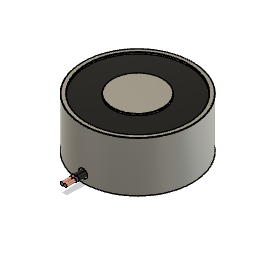
Chess_Board (Autodesk Fusion 360 archive; units mm, degrees)
design "Electromagnet_65x30"
Autodesk Fusion 360 part; units mm, degrees
sketch "Sketch1" plane through (0, 0, 0) normal (0, 1, 0) x (1, 0, 0)
  circle A0 centre (0, 0) radius 32.5
  dimension "d1" = 65
  constraint coincident A0.centre origin
  measures "d1" diameter of A0
extrude "Extrude1" add sketch "Sketch1" along normal blind 30 makes body 1
sketch "Sketch2" plane through (0, 30, 0) normal (0, 1, 0) x (-1, 0, 0)
  circle A0 centre (0, 0) radius 32.5
  circle A1 centre (0, 0) radius 15
  circle A2 centre (0, 0) radius 30
  dimension "d4" = 30
  dimension "d5" = 60
  constraint coincident A0.centre A1.centre
  measures "d4" diameter of A1
  measures "d5" diameter of A2
extrude "Extrude2" cut sketch "Sketch2" against normal blind 1 contours A2 bodies 1
fillet "Fillet1" radius 0.2 4 edges at (13.9849, 30, -5.4242) (27.9698, 30, 10.8485) (-30.3006, 30, 11.7525) (-30.3006, 0, 11.7525) on bodies 1
sketch "Sketch3" plane through (0, 0, 0) normal (0, 0, 1) x (1, 0, 0)
  circle A0 centre (0, 5) radius 2.5
  dimension "d10" = 5
  dimension "d11" = 5
  constraint vertical origin A0.centre
  measures "d10" diameter of A0
  measures "d11" distance of origin A0.centre
extrude "Extrude3" cut sketch "Sketch3" along normal blind 33 bodies 1
fillet "Fillet2" radius 0.1 1 edges at (-2.5, 5, 32.4037) on bodies 1
sketch "Sketch4" plane through (0, 0, 0) normal (0, 0, 1) x (1, 0, 0)
  circle A0 centre (0, 5) radius 2.5
  line L0 (-0.134, 5.5) -> (0.134, 5.5)
  line L1 (-0.134, 4.5) -> (0.134, 4.5)
  arc A1 (-0.134, 5.5) -> (-0.134, 4.5) centre (-1, 5) ccw
  arc A2 (0.134, 4.5) -> (0.134, 5.5) centre (1, 5) ccw
  arc A3 (0, 4.1693) -> (0, 5.8307) centre (1, 5) ccw
  arc A4 (0, 5.8307) -> (0, 4.1693) centre (-1, 5) ccw
  dimension "d16" = 2
  dimension "d17" = 2
  dimension "d18" = 5
  dimension "d19" = 1
  dimension "d20" = 0.5
  dimension "d21" = 0.5
  dimension "d22" = 0.5
  dimension "d23" = 0.3
  constraint tangent A1 A2
  constraint horizontal L0
  measures "d16" diameter of A1
  measures "d17" diameter of A2
  measures "d18" vertical distance of origin A2.centre
  measures "d19" horizontal distance of origin A1.centre
  measures "d20" distance of A1.centre L0
  measures "d21" distance of A2.centre L1
  measures "d22" distance of A1.centre L1
extrude "Extrude4" add sketch "Sketch4" along normal blind 44 contours L0 L1 A1 A2 bodies 1
extrude "Extrude5" add sketch "Sketch4" along normal blind 37 contours A3 A4 bodies 1
sketch "Sketch5" plane through (0, 0, 44) normal (0, 0, 1) x (1, 0, 0)
  arc A0 (-0.134, 5.5) -> (-0.134, 4.5) centre (-1, 5) ccw
  line L0 (-0.134, 4.5) -> (0.134, 4.5)
  arc A1 (0.134, 4.5) -> (0.134, 5.5) centre (1, 5) ccw
  line L1 (0.134, 5.5) -> (-0.134, 5.5)
  circle A2 centre (1, 5) radius 1
  circle A3 centre (-1, 5) radius 1
  constraint concentric A1 A2
  constraint concentric A0 A3
extrude "Extrude6" cut sketch "Sketch5" against normal blind 5 contours L1 A2 A3 | L0 A2 A3 bodies 1
sketch "Sketch6" plane through (0, 0, 37) normal (0, 0, 1) x (1, 0, 0)
  arc A0 (0, 5.8307) -> (0, 4.1693) centre (-1, 5) ccw
  arc A1 (0, 4.1693) -> (0, 5.8307) centre (1, 5) ccw
  arc A2 (0, 4.4321) -> (0, 5.5679) centre (1, 5) ccw
  arc A3 (0, 5.5679) -> (0, 4.4321) centre (-1, 5) ccw
  circle A4 centre (-1, 5) radius 1
  arc A5 (-0.134, 5.5) -> (-0.134, 4.5) centre (-1, 5) ccw
  line L0 (-0.134, 5.5) -> (0.134, 5.5)
  arc A6 (0.134, 4.5) -> (0.134, 5.5) centre (1, 5) ccw
  line L1 (0.134, 4.5) -> (-0.134, 4.5)
  dimension "d30" = -0.15
extrude "Extrude7" add sketch "Sketch6" along normal blind 1.5 contours A2 A3 | A4 L0 A6 L1 bodies 1
sketch "Sketch7" plane through (0, 0, 0) normal (0, -1, 0) x (1, 0, 0)
  circle A0 centre (0, 0) radius 32.3
  circle A1 centre (0, 0) radius 4
  dimension "d33" = 8
  constraint coincident A0.centre A1.centre
  measures "d33" diameter of A1
extrude "Extrude8" cut sketch "Sketch7" against normal blind 12 contours A1 bodies 1 makes body 2 at (-2.3, 4.9998, 25.7575)

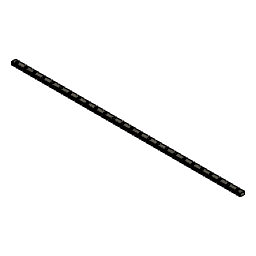
design "MGN12 Rail 650mm"
Autodesk Fusion 360 part; units mm, degrees
sketch "Sketch1" plane through (0, 0, 0) normal (1, 0, 0) x (0, 1, 0)
  line L0 (6, 0) -> (-6, 0)
  line L1 (-6, 8) -> (6, 8)
  line L2 (6, 0) -> (-6, 8) construction
  line L3 (-6, 0) -> (6, 8) construction
  line L4 (5.0369, 5.5) -> (4.7499, 5.5)
  line L5 (4.7499, 5) -> (5.0369, 5)
  line L6 (6, 8) -> (6, 6.245)
  line L7 (6, 4.255) -> (6, 0)
  arc A0 (6, 6.245) -> (5.0369, 5.5) centre (6, 5.25) ccw
  arc A1 (5.0369, 5) -> (6, 4.255) centre (6, 5.25) ccw
  line L8 (0, 8) -> (0, 0) construction
  arc A2 (-5.0369, 5.5) -> (-6, 6.245) centre (-6, 5.25) ccw
  line L9 (-5.0369, 5.5) -> (-4.7499, 5.5)
  line L10 (-4.7499, 5) -> (-5.0369, 5)
  arc A3 (-6, 4.255) -> (-5.0369, 5) centre (-6, 5.25) ccw
  line L11 (-6, 0) -> (-6, 4.255)
  line L12 (-6, 6.245) -> (-6, 8)
  arc A4 (4.7499, 5.5) -> (4.7499, 5) centre (4.7499, 5.25) ccw
  arc A5 (-4.7499, 5) -> (-4.7499, 5.5) centre (-4.7499, 5.25) ccw
  point P0 (0, 4)
  dimension "d1" = 12
  dimension "d2" = 8
  dimension "d6" = 1.99
  dimension "d23" = 1.755
  dimension "d24" = 0.5
  dimension "d25" = 0.287
  constraint perpendicular L0 L11
  constraint parallel L0 L1
  constraint parallel L6 L11
  constraint horizontal L0
  constraint coincident L2 P0
  constraint coincident L3 P0
  constraint midpoint L0 L8.end
  constraint coincident L8.end origin
  constraint perpendicular L4 L6
  constraint perpendicular L5 L6
  constraint coincident A0.centre L6
  constraint coincident L7.start L6
  constraint collinear L6 L7
  constraint coincident L5.end A0
  constraint concentric A0 A1
  constraint midpoint L1 L8.start
  constraint symmetric L7.start L8 A3.start
  constraint symmetric L6.end L8 A2.end
  constraint symmetric L4.start L8 A2.start
  constraint symmetric L5.end L8 L10.end
  constraint symmetric A0 L8 A2
  constraint symmetric A1 L8 A3
  constraint collinear L11 L12
  constraint tangent L4 A4
  constraint tangent L5 A4
  constraint horizontal A0.centre A4.centre
  constraint tangent L10 A5
  constraint tangent L9 A5
  constraint horizontal L9
  constraint horizontal L10
  constraint equal L4 L9
  measures "d1" distance of L0.start L0.end
  measures "d2" distance of L0.start L1.end
  measures "d6" diameter of A0
  measures "d23" distance of L1.end L6.end
  measures "d24" diameter of A4
  measures "d25" distance of L4.start L4.end
extrude "Extrude1" add sketch "Sketch1" along normal blind 650
chamfer "Chamfer1" distance 0.5 angle 45 16 edges at (650, 0, 8) (325, 6, 8) (650, 6, 7.1225) (650, 6, 2.1275) (650, 0, 0) (650, -6, 2.1275) (650, -6, 7.1225) (325, 6, 0) (325, -6, 0) (325, -6, 8) (0, 0, 8) (0, -6, 7.1225) (0, -6, 2.1275) (0, 6, 7.1225) (0, 6, 2.1275) (0, 0, 0)
sketch "Sketch2" plane through (0, 0, 8) normal (0, 0, 1) x (-1, 0, 0)
  line L0 (-0.5, -5.5) -> (-0.5, 5.5)
  line L1 (-0.5, 5.5) -> (-649.5, 5.5)
  line L2 (-649.5, 5.5) -> (-649.5, -5.5)
  line L3 (-649.5, -5.5) -> (-0.5, -5.5)
  line L4 (-325, -5.5) -> (-325, 5.5) construction
  circle A0 centre (-10, 0) radius 3
  dimension "d10" = 6
  dimension "d11" = 10
  constraint midpoint L3 L4.start
  constraint midpoint L1 L4.end
  measures "d10" diameter of A0
  measures "d11" distance of origin A0.centre
extrude "Extrude2" cut sketch "Sketch2" against normal blind 3.5 contours A0
sketch "Sketch3" plane through (0, 0, 4.5) normal (0, 0, 1) x (-1, 0, 0)
  circle A0 centre (-10, 0) radius 3
  circle A1 centre (-10, 0) radius 1.5
  dimension "d14" = 3
  constraint concentric A0 A1
  measures "d14" diameter of A1
extrude "Extrude3" cut sketch "Sketch3" against normal up to surface (4.5 mm away) contours A1
chamfer "Chamfer2" distance 0.5 angle 45 1 edges at (12.797, -1.0848, 8)
pattern_linear "R-Pattern1" count 26 spacing 25 along (1, 0, 0) of "Extrude2", "Extrude3", "Chamfer2"

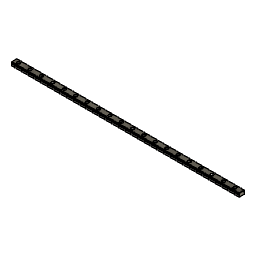
design "MGN12 Rail 500mm"
Autodesk Fusion 360 part; units mm, degrees
sketch "Sketch1" plane through (0, 0, 0) normal (1, 0, 0) x (0, 1, 0)
  line L0 (6, 0) -> (-6, 0)
  line L1 (-6, 8) -> (6, 8)
  line L2 (6, 0) -> (-6, 8) construction
  line L3 (-6, 0) -> (6, 8) construction
  line L4 (5.0369, 5.5) -> (4.7499, 5.5)
  line L5 (4.7499, 5) -> (5.0369, 5)
  line L6 (6, 8) -> (6, 6.245)
  line L7 (6, 4.255) -> (6, 0)
  arc A0 (6, 6.245) -> (5.0369, 5.5) centre (6, 5.25) ccw
  arc A1 (5.0369, 5) -> (6, 4.255) centre (6, 5.25) ccw
  line L8 (0, 8) -> (0, 0) construction
  arc A2 (-5.0369, 5.5) -> (-6, 6.245) centre (-6, 5.25) ccw
  line L9 (-5.0369, 5.5) -> (-4.7499, 5.5)
  line L10 (-4.7499, 5) -> (-5.0369, 5)
  arc A3 (-6, 4.255) -> (-5.0369, 5) centre (-6, 5.25) ccw
  line L11 (-6, 0) -> (-6, 4.255)
  line L12 (-6, 6.245) -> (-6, 8)
  arc A4 (4.7499, 5.5) -> (4.7499, 5) centre (4.7499, 5.25) ccw
  arc A5 (-4.7499, 5) -> (-4.7499, 5.5) centre (-4.7499, 5.25) ccw
  point P0 (0, 4)
  dimension "d1" = 12
  dimension "d2" = 8
  dimension "d6" = 1.99
  dimension "d23" = 1.755
  dimension "d24" = 0.5
  dimension "d25" = 0.287
  constraint perpendicular L0 L11
  constraint parallel L0 L1
  constraint parallel L6 L11
  constraint horizontal L0
  constraint coincident L2 P0
  constraint coincident L3 P0
  constraint midpoint L0 L8.end
  constraint coincident L8.end origin
  constraint perpendicular L4 L6
  constraint perpendicular L5 L6
  constraint coincident A0.centre L6
  constraint coincident L7.start L6
  constraint collinear L6 L7
  constraint coincident L5.end A0
  constraint concentric A0 A1
  constraint midpoint L1 L8.start
  constraint symmetric L7.start L8 A3.start
  constraint symmetric L6.end L8 A2.end
  constraint symmetric L4.start L8 A2.start
  constraint symmetric L5.end L8 L10.end
  constraint symmetric A0 L8 A2
  constraint symmetric A1 L8 A3
  constraint collinear L11 L12
  constraint tangent L4 A4
  constraint tangent L5 A4
  constraint horizontal A0.centre A4.centre
  constraint tangent L10 A5
  constraint tangent L9 A5
  constraint horizontal L9
  constraint horizontal L10
  constraint equal L4 L9
  measures "d1" distance of L0.start L0.end
  measures "d2" distance of L0.start L1.end
  measures "d6" diameter of A0
  measures "d23" distance of L1.end L6.end
  measures "d24" diameter of A4
  measures "d25" distance of L4.start L4.end
extrude "Extrude1" add sketch "Sketch1" along normal blind 500
chamfer "Chamfer1" distance 0.5 angle 45 16 edges at (500, 0, 8) (250, 6, 8) (500, 6, 7.1225) (500, 6, 2.1275) (500, 0, 0) (500, -6, 2.1275) (500, -6, 7.1225) (250, 6, 0) (250, -6, 0) (250, -6, 8) (0, 0, 8) (0, -6, 7.1225) (0, -6, 2.1275) (0, 6, 7.1225) (0, 6, 2.1275) (0, 0, 0)
sketch "Sketch2" plane through (0, 0, 8) normal (0, 0, 1) x (-1, 0, 0)
  line L0 (-0.5, -5.5) -> (-0.5, 5.5)
  line L1 (-0.5, 5.5) -> (-499.5, 5.5)
  line L2 (-499.5, 5.5) -> (-499.5, -5.5)
  line L3 (-499.5, -5.5) -> (-0.5, -5.5)
  line L4 (-250, -5.5) -> (-250, 5.5) construction
  circle A0 centre (-10, 0) radius 3
  dimension "d10" = 6
  dimension "d11" = 10
  constraint midpoint L3 L4.start
  constraint midpoint L1 L4.end
  measures "d10" diameter of A0
  measures "d11" distance of origin A0.centre
extrude "Extrude2" cut sketch "Sketch2" against normal blind 3.5 contours A0
sketch "Sketch3" plane through (0, 0, 4.5) normal (0, 0, 1) x (-1, 0, 0)
  circle A0 centre (-10, 0) radius 3
  circle A1 centre (-10, 0) radius 1.5
  dimension "d14" = 3
  constraint concentric A0 A1
  measures "d14" diameter of A1
extrude "Extrude3" cut sketch "Sketch3" against normal up to surface (4.5 mm away) contours A1
chamfer "Chamfer2" distance 0.5 angle 45 1 edges at (12.797, -1.0848, 8)
pattern_linear "R-Pattern1" count 20 spacing 25 along (1, 0, 0) of "Extrude2", "Extrude3", "Chamfer2"
